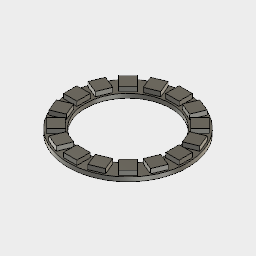
1463 16x NeoPixel Ring (Autodesk Fusion 360 design; units mm, degrees)
Autodesk Fusion 360 part; units mm, degrees
sketch "PCB" plane through (0, 0, 0) normal (0, 0, 1) x (1, 0, 0)
  circle A0 centre (0, 0) radius 15.875
  circle A1 centre (0, 0) radius 22.225
  dimension "d1" = 31.75
  dimension "d2" = 44.45
  measures "d1" diameter of A0
  measures "d2" diameter of A1
extrude "Extrude1" add sketch "PCB" along normal blind 1.6 makes body 1
sketch "LEDs" plane through (0, 0, 1.6) normal (0, 0, 1) x (-1, 0, 0)
  circle A0 centre (0, 0) radius 15.875
  circle A1 centre (0, 0) radius 22.225
  line L0 (-2.5013, -16.4993) -> (2.4987, -16.4993)
  line L1 (2.4987, -16.4993) -> (2.4987, -21.4993)
  line L2 (2.4987, -21.4993) -> (-2.5013, -21.4993)
  line L3 (-2.5013, -21.4993) -> (-2.5013, -16.4993)
  line L4 (-2.5013, -16.4993) -> (2.4987, -21.4993) construction
  line L5 (2.4987, -16.4993) -> (-2.5013, -21.4993) construction
  line L6 (10.5359, -18.9066) -> (5.9165, -20.82)
  line L7 (8.6225, -14.2872) -> (10.5359, -18.9066)
  line L8 (5.9165, -20.82) -> (4.0031, -16.2006)
  line L9 (4.0031, -16.2006) -> (8.6225, -14.2872)
  line L10 (16.9691, -13.4355) -> (13.4336, -16.971)
  line L11 (13.4336, -9.8999) -> (16.9691, -13.4355)
  line L12 (13.4336, -16.971) -> (9.898, -13.4355)
  line L13 (9.898, -13.4355) -> (13.4336, -9.8999)
  line L14 (20.8189, -5.919) -> (18.9055, -10.5384)
  line L15 (16.1996, -4.0055) -> (20.8189, -5.919)
  line L16 (18.9055, -10.5384) -> (14.2861, -8.6249)
  line L17 (14.2861, -8.6249) -> (16.1996, -4.0055)
  line L18 (21.4993, 2.4987) -> (21.4993, -2.5013)
  line L19 (16.4993, 2.4987) -> (21.4993, 2.4987)
  line L20 (21.4993, -2.5013) -> (16.4993, -2.5013)
  line L21 (16.4993, -2.5013) -> (16.4993, 2.4987)
  line L22 (18.9066, 10.5359) -> (20.82, 5.9165)
  line L23 (14.2872, 8.6225) -> (18.9066, 10.5359)
  line L24 (20.82, 5.9165) -> (16.2006, 4.0031)
  line L25 (16.2006, 4.0031) -> (14.2872, 8.6225)
  line L26 (13.4355, 16.9691) -> (16.971, 13.4336)
  line L27 (9.8999, 13.4336) -> (13.4355, 16.9691)
  line L28 (16.971, 13.4336) -> (13.4355, 9.898)
  line L29 (13.4355, 9.898) -> (9.8999, 13.4336)
  line L30 (5.919, 20.8189) -> (10.5384, 18.9055)
  line L31 (4.0055, 16.1996) -> (5.919, 20.8189)
  line L32 (10.5384, 18.9055) -> (8.6249, 14.2861)
  line L33 (8.6249, 14.2861) -> (4.0055, 16.1996)
  line L34 (-2.4987, 21.4993) -> (2.5013, 21.4993)
  line L35 (-2.4987, 16.4993) -> (-2.4987, 21.4993)
  line L36 (2.5013, 21.4993) -> (2.5013, 16.4993)
  line L37 (2.5013, 16.4993) -> (-2.4987, 16.4993)
  line L38 (-10.5359, 18.9066) -> (-5.9165, 20.82)
  line L39 (-8.6225, 14.2872) -> (-10.5359, 18.9066)
  line L40 (-5.9165, 20.82) -> (-4.0031, 16.2006)
  line L41 (-4.0031, 16.2006) -> (-8.6225, 14.2872)
  line L42 (-16.9691, 13.4355) -> (-13.4336, 16.971)
  line L43 (-13.4336, 9.8999) -> (-16.9691, 13.4355)
  line L44 (-13.4336, 16.971) -> (-9.898, 13.4355)
  line L45 (-9.898, 13.4355) -> (-13.4336, 9.8999)
  line L46 (-20.8189, 5.919) -> (-18.9055, 10.5384)
  line L47 (-16.1996, 4.0055) -> (-20.8189, 5.919)
  line L48 (-18.9055, 10.5384) -> (-14.2861, 8.6249)
  line L49 (-14.2861, 8.6249) -> (-16.1996, 4.0055)
  line L50 (-21.4993, -2.4987) -> (-21.4993, 2.5013)
  line L51 (-16.4993, -2.4987) -> (-21.4993, -2.4987)
  line L52 (-21.4993, 2.5013) -> (-16.4993, 2.5013)
  line L53 (-16.4993, 2.5013) -> (-16.4993, -2.4987)
  line L54 (-18.9066, -10.5359) -> (-20.82, -5.9165)
  line L55 (-14.2872, -8.6225) -> (-18.9066, -10.5359)
  line L56 (-20.82, -5.9165) -> (-16.2006, -4.0031)
  line L57 (-16.2006, -4.0031) -> (-14.2872, -8.6225)
  line L58 (-13.4355, -16.9691) -> (-16.971, -13.4336)
  line L59 (-9.8999, -13.4336) -> (-13.4355, -16.9691)
  line L60 (-16.971, -13.4336) -> (-13.4355, -9.898)
  line L61 (-13.4355, -9.898) -> (-9.8999, -13.4336)
  line L62 (-5.919, -20.8189) -> (-10.5384, -18.9055)
  line L63 (-4.0055, -16.1996) -> (-5.919, -20.8189)
  line L64 (-10.5384, -18.9055) -> (-8.6249, -14.2861)
  line L65 (-8.6249, -14.2861) -> (-4.0055, -16.1996)
  point P0 (-0.0013, -18.9993)
  dimension "d5" = 5
  dimension "d6" = 5
  dimension "d8" = 360
  measures "d5" distance of L1.end L2.end
  measures "d6" distance of L0.end L1.end
extrude "Extrude2" add sketch "LEDs" along normal blind 1.7 separate body contours L0 L1 L2 L3 | L6 L7 L8 L9 | L10 L11 L12 L13 | L14 L15 L16 L17 | L18 L19 L20 L21 | L22 L23 L24 L25 | L26 L27 L28 L29 | L30 L31 L32 L33 | L34 L35 L36 L37 | L38 L39 L40 L41 | L42 L43 L44 L45 | L46 L47 L48 L49 | L50 L51 L52 L53 | L54 L55 L56 L57 | L58 L59 L60 L61 | L62 L63 L64 L65 makes body 2 at (13.4336, -12.257, 1.6) makes body 3 at (-6.1832, -17.1015, 1.6) makes body 4 at (-16.4648, -7.7205, 1.6) makes body 5 at (-7.7205, 16.4648, 1.6) makes body 6 at (-0.832, 18.166, 1.6) makes body 7 at (6.821, 18.6413, 1.6) makes body 8 at (18.6424, 6.8185, 1.6) makes body 9 at (7.7205, -16.4648, 1.6) makes body 10 at (17.1015, -6.1832, 1.6) makes body 11 at (-12.257, -13.4336, 1.6) makes body 12 at (-18.166, -0.832, 1.6) makes body 13 at (-13.4336, 12.257, 1.6) makes body 14 at (-18.0035, 8.3608, 1.6) makes body 15 at (13.4355, 14.6121, 1.6) makes body 16 at (19.8326, -0.8347, 1.6) makes body 17 at (0.832, -18.166, 1.6)
sketch "mount tester" plane through (0, 0, 0) normal (0, 0, 1) x (1, 0, 0)
  circle A0 centre (0, 0) radius 25.5
  circle A1 centre (0, 0) radius 22.225
  circle A2 centre (0, 0) radius 15.875
  circle A3 centre (0, 0) radius 23.425
  circle A4 centre (0, 0) radius 14.675
  circle A5 centre (0, 0) radius 22.425
  circle A6 centre (0, 0) radius 15.675
  dimension "d11" = 51
  dimension "d12" = 0.2
  dimension "d13" = 0.2
  dimension "d18" = 1
  dimension "d19" = 1
  measures "d11" diameter of A0
  measures "d18" distance of A3 A5
  measures "d19" distance of A4 A6
extrude "Extrude3" add sketch "mount tester" against normal blind 1 separate body contours A0 | A1 | A2 | A3 | A5 | A6 makes body 18
extrude "Extrude4" add sketch "mount tester" along normal blind 3.5 contours A3 | A6 bodies 18
chamfer "Chamfer1" distance 1 angle 45 1 edges at (-23.7743, 9.2212, -1) on bodies 18
hidden bodies 18
